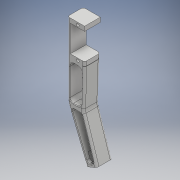
# Autodesk Inventor part: noga
Saved by Autodesk Inventor 2018 (Build 220112000, 112)
## iProperties
Created: 2020-10-02
Part Number: noga
Material: Ogólny
Document SubType Name: Modeling
Designer: Raven
Density: 1 g/cm^3
Appearance: Domyślna
Author: Raven
Autodesk Inventor part; units mm, degrees
ref_plane "YZ Plane" through (0, 0, 0) normal (1, 0, 0) x (0, 1, 0)
ref_plane "XZ Plane" through (0, 0, 0) normal (0, 1, 0) x (-1, 0, 0)
ref_plane "XY Plane" through (0, 0, 0) normal (0, 0, 1) x (1, 0, 0)
sketch "Szkic1" plane through (0, 0, 0) normal (0, 1, 0) x (-1, 0, 0)
  line L0 (0, 0) -> (12.2, 0) construction
  line L1 (12.2, 0) -> (15.2, 0) construction
  line L2 (0, 0) -> (0, -4) construction
  line L3 (0, -4) -> (12.7, -4) construction
  line L4 (12.7, -4) -> (12.7, -27.6) construction
  line L5 (12.7, -27.6) -> (0, -27.6) construction
  line L6 (0, -27.6) -> (0, -31.6) construction
  line L7 (0, -31.6) -> (12.7, -31.6) construction
  line L8 (15.2, 0) -> (15.2, -31.6) construction
  line L9 (15.2, -31.6) -> (12.7, -31.6) construction
  line L10 (6.1, 0) -> (6.1, -2.1) construction
  circle A0 centre (6.1, -2.1) radius 1.25 construction
  line L11 (6.1, 0) -> (6.6, 0) construction
  line L12 (12.7, -15.8) -> (0, -15.8) construction
  circle A1 centre (6.1, -29.5) radius 1.25 construction
  line L13 (15.2, -31.6) -> (15.2, -66.6) construction
  line L14 (15.2, -66.6) -> (1.2, -66.6) construction
  line L15 (0, -31.6) -> (1.2, -66.6) construction
  line L16 (1.2, -66.6) -> (-10.8, -66.6) construction
  line L17 (-10.8, -66.6) -> (-10.8, -103.6) construction
  line L18 (1.2, -66.6) -> (-10.8, -103.6) construction
  line L19 (-10.8, -103.6) -> (-10.8, -108.6) construction
  line L20 (-10.8, -108.6) -> (-1.8, -108.6) construction
  line L21 (-1.8, -108.6) -> (15.2, -66.6) construction
  line L22 (-10.8, -103.6) -> (-1.328, -107.4339) construction
  line L23 (12.7, -4) -> (0, -4)
  line L24 (0, -4) -> (0, 0)
  line L25 (0, 0) -> (15.2, 0)
  line L26 (15.2, 0) -> (15.2, -66.6)
  line L27 (0, -31.6) -> (1.2, -66.6)
  line L28 (1.2, -66.6) -> (-10.8, -103.6)
  line L29 (-10.8, -103.6) -> (-1.328, -107.4339)
  line L30 (15.2, -66.6) -> (-1.328, -107.4339)
  circle A2 centre (6.1, -29.5) radius 1.25
  circle A3 centre (6.1, -2.1) radius 1.25
  line L31 (12.7, -4) -> (12.7, -27.6)
  line L32 (12.7, -27.6) -> (0, -27.6)
  line L33 (0, -27.6) -> (0, -31.6)
  dimension "d1" = 12.2
  dimension "d2" = 3
  dimension "d5" = 4
  dimension "d8" = 31.6
  dimension "d14" = 2.1
  dimension "d15" = 2.5
  dimension "d18" = 35
  dimension "d19" = 14
  dimension "d20" = 12
  dimension "d21" = 37
  dimension "d22" = 5
  dimension "d23" = 9
  dimension "d86" = 2.1
  dimension "d87" = 4
  dimension "d88" = 23.6
  dimension "d89" = 12.7
  constraints: 68 end point, 10 collinear, 8 perpendicular, 6 vertical, 4 centre point, 4 horizontal, 4 point on line, 3 coincident, 2 concentric, 2 midpoint, 1 symmetric about line, 1 other
  measures "d1" distance of L0.start L0.end
  measures "d2" distance of L0.end L1.end
  measures "d5" distance of L0.start L2.end
  measures "d8" distance of L6.end L0.start
  measures "d14" distance of L10.start L10.end
  measures "d15" diameter of A0
  measures "d18" distance of L8.end L13.end
  measures "d19" distance of L13.end L14.end
  measures "d20" distance of L14.end L16.end
  measures "d21" distance of L16.end L17.end
  measures "d22" distance of L17.end L19.end
  measures "d23" distance of L19.end L20.end
  measures "d86" distance from line of L7 A1.centre
  measures "d87" distance of L5.end L6.end
  measures "d88" distance of L3.end L4.end
  measures "d89" distance of L2.end L3.end
extrude "Wyciągnięcie proste1" add sketch "Szkic1" along normal blind 14
sketch "Szkic2" plane through (0, 14, 0) normal (0, 1, 0) x (1, 0, 0)
  line L0 (0, 27.6) -> (0, 31.6) construction
  line L1 (0, 31.6) -> (-15.2, 31.6) construction
  line L2 (-15.2, 31.6) -> (-15.2, 66.6) construction
  line L3 (0, 31.6) -> (-1.2, 66.6) construction
  line L4 (-15.2, 66.6) -> (-1.2, 66.6) construction
  line L5 (-1.2, 66.6) -> (0, 31.6) construction
  line L6 (-13.2, 64.6) -> (-13.2, 33.6) construction
  line L7 (-13.2, 33.6) -> (-2.0697, 33.6) construction
  line L8 (-2.0697, 33.6) -> (-3.1326, 64.6) construction
  line L9 (-3.1326, 64.6) -> (-13.2, 64.6) construction
  line L10 (1.328, 107.4339) -> (-15.2, 66.6) construction
  line L11 (-15.2, 66.6) -> (1.328, 107.4339) construction
  line L12 (1.328, 107.4339) -> (7.3944, 104.9785) construction
  line L13 (7.3944, 104.9785) -> (-1.2, 66.6) construction
  line L14 (-13.2, 33.6) -> (-13.2, 64.6)
  line L15 (-13.2, 64.6) -> (-3.1326, 64.6)
  line L16 (-3.1326, 64.6) -> (-2.0697, 33.6)
  line L17 (-2.0697, 33.6) -> (-13.2, 33.6)
  point P0 (0, 0)
  dimension "d26" = 15.2
  dimension "d27" = 2
  constraints: 30 end point, 6 collinear, 1 horizontal, 1 perpendicular, 1 point on line, 3 other
  measures "d26" distance of L0.end L1.end
  measures "d27" distance between parallel lines of L2 L6
extrude "Wyciągnięcie proste2" cut sketch "Szkic2" against normal blind 14
sketch "Szkic3" plane through (0, 14, 0) normal (0, 1, 0) x (1, 0, 0)
  line L0 (1.328, 107.4339) -> (-15.2, 66.6) construction
  line L1 (-1.2, 66.6) -> (-15.2, 66.6) construction
  line L2 (-15.2, 66.6) -> (1.328, 107.4339) construction
  line L3 (-1.2, 66.6) -> (10.8, 103.6) construction
  line L4 (1.328, 107.4339) -> (10.8, 103.6) construction
  line L5 (10.8, 103.6) -> (-1.2, 66.6) construction
  line L6 (-12.2329, 68.6) -> (-2.6539, 68.6) construction
  line L7 (-2.6539, 68.6) -> (8.3229, 102.445) construction
  line L8 (8.3229, 102.445) -> (2.4315, 104.8296) construction
  line L9 (2.4315, 104.8296) -> (-12.2329, 68.6) construction
  line L10 (-12.2329, 68.6) -> (2.4315, 104.8296)
  line L11 (8.3229, 102.445) -> (2.4315, 104.8296)
  line L12 (8.3229, 102.445) -> (-2.6539, 68.6)
  line L13 (-2.6539, 68.6) -> (-12.2329, 68.6)
  point P0 (0, 0)
  dimension "d30" = 2
  constraints: 24 end point, 5 collinear, 2 perpendicular, 1 horizontal, 3 other
  measures "d30" distance between parallel lines of L1 L6
extrude "Wyciągnięcie proste3" cut sketch "Szkic3" against normal blind 14
fillet "Zaokrąglenie1" radius 10 1 edges at (-15.2, 7, -66.6)
fillet "Zaokrąglenie2" radius 10 1 edges at (-1.2, 7, -66.6)
fillet "Zaokrąglenie3" radius 10 1 edges at (0, 7, -31.6)
fillet "Zaokrąglenie4" radius 2 1 edges at (-12.2329, 7, -68.6)
fillet "Zaokrąglenie5" radius 2 1 edges at (-2.6539, 7, -68.6)
fillet "Zaokrąglenie8" radius 4 2 edges at (-13.2, 7, -33.6) (-2.0697, 7, -33.6)
fillet "Zaokrąglenie9" radius 3 2 edges at (-13.2, 7, -64.6) (-3.1326, 7, -64.6)
fillet "Zaokrąglenie12" radius 2.6 2 edges at (8.3229, 7, -102.445) (2.4315, 7, -104.8296)
fillet "Zaokrąglenie10" radius 2 14 edges at (-15.0157, 14, -66.5641) (-6.5707, 14, -87.9194) (-15.2, 14, -32.3265) (-15.0157, 0, -66.5641) (-6.5707, 0, -87.9194) (-15.2, 0, -32.3265) (-1.0483, 14, -66.5787) (5.0711, 14, -85.9358) (-0.0015, 14, -31.6) (-0.5728, 14, -48.3075) (-1.0483, 0, -66.5787) (5.0711, 0, -85.9358) (-0.0015, 0, -31.6) (-0.5728, 0, -48.3075)
fillet "Zaokrąglenie11" radius 0.5 26 edges at (-12.0284, 0, -34.7716) (-7.7046, 0, -33.6) (-3.3328, 0, -34.8205) (-2.6224, 0, -49.7199) (-3.9468, 0, -63.7574) (-8.1158, 0, -64.6) (-12.3213, 0, -63.7213) (-13.2, 0, -49.6) (-12.3213, 14, -63.7213) (-8.1158, 14, -64.6) (-3.9468, 14, -63.7574) (-2.6224, 14, -49.7199) (-3.3328, 14, -34.8205) (-7.7046, 14, -33.6) (-12.0284, 14, -34.7716) (-13.2, 14, -49.6) (2.6852, 14, -85.0622) (-2.9318, 14, -68.9823) (-6.6868, 14, -68.6) (-10.9241, 14, -69.4821) (-4.8318, 14, -86.885) (-4.8318, 0, -86.885) (-10.9241, 0, -69.4821) (-6.6868, 0, -68.6) (-2.9318, 0, -68.9823) (2.6852, 0, -85.0622)
sketch "Szkic4" plane through (1.328, 2, -107.4339) normal (0.3751928, 0, -0.9269468) x (-0.9269468, 0, -0.3751928)
  line L0 (-8.2134, -2) -> (-2, -2) construction
  line L1 (-4.6, 12) -> (-2, 12) construction
  line L2 (0, 0) -> (0, 10) construction
  line L3 (-10.2185, 0) -> (-10.2185, 10) construction
  line L4 (-5.1067, -2) -> (-5.1067, 12) construction
  line L5 (-26.8417, 12) -> (-2.5844, 12) construction
  line L6 (-5.1067, -2) -> (8.8933, -2) construction
  line L7 (0, 10) -> (0, 0) construction
  line L8 (0, 5) -> (-10.2185, 5) construction
  line L9 (-5.1092, 5) -> (-1.3592, 5) construction
  line L10 (-1.3592, 5) -> (-1.3592, 8.75) construction
  line L11 (-1.3592, 8.75) -> (-8.8592, 8.75)
  line L12 (-8.8592, 8.75) -> (-8.8592, 1.25)
  line L13 (-8.8592, 1.25) -> (-1.3592, 1.25)
  line L14 (-1.3592, 1.25) -> (-1.3592, 8.75)
  point P0 (-39.0774, -2)
  point P1 (-9.1909, 13)
  point P2 (-2.5844, 12)
  point P3 (-9.1909, 12)
  dimension "d66" = 90
  dimension "d67" = 3.75
  dimension "d68" = 3.75
  dimension "d69" = 7.5
  dimension "d70" = 7.5
  constraints: 18 end point, 4 midpoint, 2 horizontal, 2 parallel, 2 perpendicular, 1 point on line, 1 vertical, 3 other
  measures "d66" angle of L6 L4
  measures "d67" distance of L9.start L9.end
  measures "d68" distance of L9.end L10.end
  measures "d69" distance of L13.end L12.end
  measures "d70" distance of L12.end L11.end
extrude "Wyciągnięcie proste4" cut sketch "Szkic4" against normal blind 9
sketch "Szkic8" plane through (1.328, 2, -107.4339) normal (0.3751928, 0, -0.9269468) x (-0.9269468, 0, -0.3751928)
  line L0 (-8.8592, 8.75) -> (-1.3592, 8.75) projected
  line L1 (-5.1092, 8.75) -> (-5.1092, 1.25) construction
  line L2 (-8.2134, 12) -> (-2, 12) construction
  line L3 (-8.2134, -2) -> (-2, -2) construction
  line L4 (-5.1092, 8.75) -> (-5.1092, 12) construction
  line L5 (-26.8417, 12) -> (-2.5844, 12) construction
  line L6 (-5.1092, 8.75) -> (-3.6092, 8.75) construction
  line L7 (-3.6092, 8.75) -> (-6.6092, 8.75)
  line L8 (-6.6092, 8.75) -> (-6.6092, 10.25)
  line L9 (-6.6092, 10.25) -> (-3.6092, 10.25)
  line L10 (-3.6092, 10.25) -> (-3.6092, 8.75)
  line L11 (-3.6092, 8.75) -> (-3.6092, 1.25) construction
  line L12 (-1.3592, 1.25) -> (-8.8592, 1.25) construction
  line L13 (-3.6092, 1.25) -> (-6.6092, 1.25)
  line L14 (-6.6092, 1.25) -> (-6.6092, -0.25)
  line L15 (-6.6092, -0.25) -> (-3.6092, -0.25)
  line L16 (-3.6092, -0.25) -> (-3.6092, 1.25)
  point P0 (-39.0774, -2)
  dimension "d77" = 7.5
  dimension "d78" = 1.5
  dimension "d79" = 3
  dimension "d80" = 1.5
  dimension "d81" = 3
  dimension "d82" = 1.5
  constraints: 24 end point, 4 parallel, 3 perpendicular, 3 point on line, 2 horizontal, 2 vertical, 1 midpoint
  measures "d77" distance of L1.start L1.end
  measures "d78" distance of L1.start L6.end
  measures "d79" distance of L8.end L9.end
  measures "d80" distance of L7.end L8.end
  measures "d81" distance of L15.end L14.end
  measures "d82" distance of L14.end L13.end
extrude "Wyciągnięcie proste8" cut sketch "Szkic8" against normal blind 9
sketch "Szkic6" plane through (-4.1078, 0.5, -68.6) normal (0, 0, -1) x (-1, 0, 0)
  line L0 (5.1579, 13) -> (5.1579, 0) projected
  line L1 (0, 0) -> (0, 13) projected
  line L2 (5.1579, 6.5) -> (0, 6.5) construction
  circle A0 centre (2.5789, 6.5) radius 1.5
  point P0 (-4.1078, -0.5)
  point P1 (0.8707, 1)
  point P2 (-2, 1)
  point P3 (4.4309, 13)
  point P4 (4.4309, -1)
  point P5 (-0.727, -1)
  point P6 (-0.727, 13)
  dimension "d58" = 3
  constraints: 2 end point, 1 centre point, 1 midpoint, 4 other
  measures "d58" diameter of A0
extrude "Wyciągnięcie proste6" cut sketch "Szkic6" against normal blind 7
